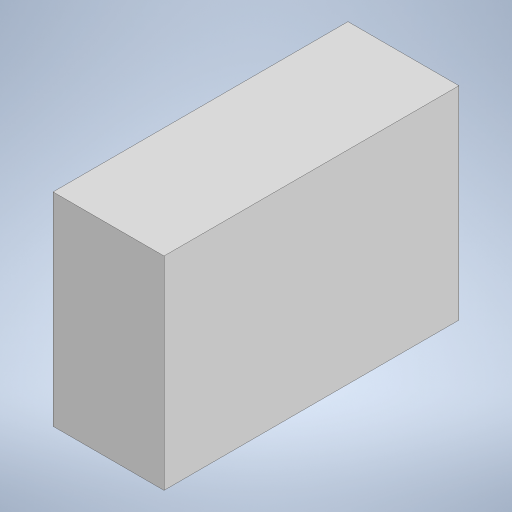
# Autodesk Inventor part: parameter checker
Saved by Autodesk Inventor 2023 (Build 270158000, 158)
## iProperties
Created: 2023-01-16
Part Number: parameter checker
Material: Generic
Document SubType Name: Modeling
Designer: Gabriel - T3 CAD
Density: 1 g/cm^3
Appearance: Default
Author: Gabriel - T3 CAD
Autodesk Inventor part; units mm, degrees
ref_plane "YZ Plane" through (0, 0, 0) normal (1, 0, 0) x (0, 1, 0)
ref_plane "XZ Plane" through (0, 0, 0) normal (0, 1, 0) x (-1, 0, 0)
ref_plane "XY Plane" through (0, 0, 0) normal (0, 0, 1) x (1, 0, 0)
sketch "Sketch1" plane through (0, 0, 0) normal (0, 1, 0) x (-1, 0, 0)
  line L0 (0, 0) -> (635, 0)
  line L1 (635, 0) -> (635, 889)
  line L2 (635, 889) -> (0, 889)
  line L3 (0, 889) -> (0, 0)
  line L4 (-127, 0) -> (762, 0)
  line L5 (762, 0) -> (762, 1016)
  line L6 (762, 1016) -> (-127, 1016)
  line L7 (-127, 1016) -> (-127, 0)
  line L8 (0, 0) -> (635, 0)
  line L9 (635, 0) -> (635, -1219.2)
  line L10 (635, -1219.2) -> (0, -1219.2)
  line L11 (0, -1219.2) -> (0, 0)
  line L12 (-127, 0) -> (762, 0)
  line L13 (762, 0) -> (762, -1346.2)
  line L14 (762, -1346.2) -> (-127, -1346.2)
  line L15 (-127, -1346.2) -> (-127, 0)
  point P0 (762, 0)
  dimension "d0" = 635
  dimension "d1" = 889
  dimension "d2" = 889
  dimension "d3" = 1016
  dimension "d4" = 127
  dimension "d9" = 635
  dimension "d10" = 1219.2
  dimension "d11" = 889
  dimension "d12" = 1346.2
  constraints: 32 end point, 8 parallel, 4 horizontal, 4 perpendicular, 1 point on line
  measures "d0" distance of L2.end L1.end
  measures "d1" distance of L1.end L0.end
  measures "d2" distance of L6.end L5.end
  measures "d3" distance of L5.end L4.end
  measures "d4" distance between parallel lines of L3 L7
  measures "d9" distance of L9.end L10.end
  measures "d10" distance of L8.end L9.end
  measures "d11" distance of L13.end L14.end
  measures "d12" distance of L12.end L13.end
extrude "Extrusion1" add sketch "Sketch1" along normal mid plane 1625.6
extrude "Extrusion2" cut sketch "Sketch1" along normal mid plane 1371.6 contours L3 L2 L1 L0 | L0 L9 L10 L11
body "Solid1"
